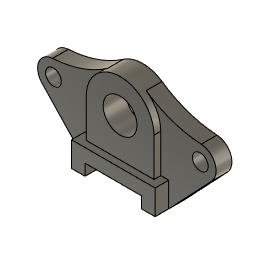
NCV-12 v3 (Autodesk Fusion 360 design; units mm, degrees)
Autodesk Fusion 360 part; units mm, degrees
sketch "Sketch1" plane through (0, 0, 0) normal (0, 1, 0) x (1, 0, 0)
  line L0 (-37, 0) -> (37, 0)
  line L1 (37, 0) -> (37, 22)
  line L2 (37, 22) -> (25, 22)
  line L3 (25, 22) -> (25, 12)
  line L4 (25, 12) -> (-25, 12)
  line L5 (-25, 12) -> (-25, 22)
  line L6 (-25, 22) -> (-37, 22)
  line L7 (-37, 22) -> (-37, 0)
  circle A0 centre (0, -34) radius 15
  circle A1 centre (0, -34) radius 30
  line L8 (-30, 0) -> (-30, -34)
  line L9 (30, 0) -> (30, -34)
  circle A2 centre (65, -28) radius 7
  circle A3 centre (65, -28) radius 14
  line L10 (37, 22) -> (75.1738, -18.3827)
  arc A4 (65.7795, -41.9783) -> (17.0566, -58.6794) centre (71.069, -136.8309) ccw
  dimension "d1" = 25
  dimension "d2" = 25
  dimension "d3" = 37
  dimension "d4" = 37
  dimension "d5" = 22
  dimension "d6" = 22
  dimension "d7" = 12
  dimension "d8" = 12
  dimension "d9" = 30
  dimension "d10" = 34
  dimension "d11" = 37
  dimension "d12" = 60
  dimension "d13" = 14
  dimension "d14" = 28
  dimension "d15" = 65
  dimension "d16" = 28
  dimension "d17" = 190
  constraint horizontal L0
  constraint vertical L1
  constraint horizontal L2
  constraint vertical L3
  constraint horizontal L4
  constraint vertical L5
  constraint horizontal L6
  constraint vertical L7
  constraint concentric A0 A1
  constraint coincident L0 L8.start
  constraint coincident L0 L9.start
  constraint vertical L8
  constraint vertical L9
  constraint tangent A1 L8
  constraint tangent A1 L9
  constraint coincident A1 L8.end
  constraint coincident A1 L9.end
  constraint concentric A2 A3
  constraint tangent A3 L10
  constraint coincident A3 L10.end
  constraint tangent A3 A4
  constraint tangent A1 A4
  constraint coincident A1 A4.end
  constraint coincident A3 A4.start
  measures "d1" horizontal distance of origin L2.end
  measures "d2" horizontal distance of origin L5.end
  measures "d3" horizontal distance of origin L1.end
  measures "d4" horizontal distance of origin L6.end
  measures "d5" vertical distance of origin L6.end
  measures "d6" vertical distance of origin L1.end
  measures "d7" vertical distance of origin L4.end
  measures "d8" vertical distance of L0.start L4.end
  measures "d9" diameter of A0
  measures "d10" vertical distance of origin A0.centre
  measures "d11" horizontal distance of L0.end A0.centre
  measures "d12" diameter of A1
  measures "d13" diameter of A2
  measures "d14" diameter of A3
  measures "d15" horizontal distance of origin A2.centre
  measures "d16" vertical distance of origin A2.centre
  measures "d17" diameter of A4
extrude "Extrude1" add sketch "Sketch1" against normal blind 26 contours L0 L1 L2 L3 L4 L5 L6 L7
extrude "Extrude2" add sketch "Sketch1" against normal blind 20 contours L0 A1 L8 L9 | A1
extrude "Extrude3" add sketch "Sketch1" against normal blind 14 contours L0 L1 A1 L9 A3 L10 A4 | A3
mirror "Mirror1" about plane through (0, 0, 0) normal (1, 0, 0) of "Extrude3"
equation "d1 = ( 50 / 2 ) * 1 mm"
equation "d2 = d1"
equation "d3 = d1 + 12 mm"
equation "d4 = d3"
equation "d7 = d6 - 10 mm"
equation "d8 = d7"
equation "d11 = d3"
equation "d14 = ( 14 * 2 ) * 1 mm"
equation "d15 = ( 130 / 2 ) * 1 mm"
equation "d16 = 50 mm - 22 mm"
equation "d17 = ( 95 * 2 ) * 1 mm"
